Autodesk Fusion 360 part; units mm, degrees
(part 4 of 5)
sketch "Sketch2" plane through (0, 0, 0) normal (0, 0, 1) x (1, 0, 0) in component "spoilboard v12"
  arc A0 (1101.5761, 607.1637) -> (1101.5763, 647.1637) centre (1101.5762, 627.1637) ccw
  arc A1 (117.6237, 647.1637) -> (117.6239, 607.1637) centre (117.6238, 627.1637) ccw
  arc A2 (916.5761, 607.1637) -> (916.5763, 647.1637) centre (916.5762, 627.1637) ccw
  arc A3 (1036.0507, 647.1575) -> (1035.5361, 607.1642) centre (1036.0526, 627.1575) ccw
  line L0 (1016.0526, 627.1635) -> (1121.5762, 627.1635) construction
  line L1 (936.5762, 627.1635) -> (1016.0526, 627.1635) construction
  circle A4 centre (976.3144, 627.1635) radius 1.5875
  arc A5 (368.6639, 607.1642) -> (368.1493, 647.1575) centre (368.1474, 627.1575) ccw
  arc A6 (487.6237, 647.1637) -> (487.6239, 607.1637) centre (487.6238, 627.1637) ccw
  line L2 (97.6238, 627.1635) -> (388.1474, 627.1635) construction
  line L3 (467.6238, 627.1635) -> (936.5762, 627.1635) construction
  line L4 (388.1474, 627.1635) -> (467.6238, 627.1635) construction
  circle A7 centre (427.8856, 627.1635) radius 1.5875
  circle A8 centre (34.29, 1220) radius 17.145
  circle A9 centre (1184.91, 1220) radius 17.145
  circle A10 centre (897.255, 1220) radius 17.145
  circle A11 centre (609.6, 1220) radius 17.145
  line L5 (34.29, 1220) -> (626.745, 1220) construction
  line L6 (880.11, 1220) -> (1184.91, 1220) construction
  line L7 (626.745, 1220) -> (880.11, 1220) construction
  circle A12 centre (753.4275, 1220) radius 1.5875
  arc A13 (33.02, 1953.1525) -> (33.02, 1913.1525) centre (33.02, 1933.1525) ccw
  arc A14 (1186.18, 1913.1525) -> (1186.18, 1953.1525) centre (1186.18, 1933.1525) ccw
  arc A15 (461.4333, 1913.1525) -> (461.4333, 1953.1525) centre (461.4333, 1933.1525) ccw
  arc A16 (576.58, 1953.1525) -> (576.58, 1913.1525) centre (576.58, 1933.1525) ccw
  line L8 (33.02, 1933.1525) -> (481.4333, 1933.1525) construction
  line L9 (556.58, 1933.1525) -> (1186.18, 1933.1525) construction
  line L10 (481.4333, 1933.1525) -> (556.58, 1933.1525) construction
  circle A17 centre (519.0067, 1933.1525) radius 1.5875
  circle A18 centre (753.4275, 1220) radius 6
  circle A19 centre (976.3144, 627.1635) radius 6
  circle A20 centre (427.8856, 627.1635) radius 6
  circle A21 centre (519.0067, 1933.1525) radius 6
  arc A22 (117.6237, 1847.1637) -> (117.6239, 1807.1637) centre (117.6238, 1827.1637) ccw
  arc A23 (1101.5761, 1807.1637) -> (1101.5763, 1847.1637) centre (1101.5762, 1827.1637) ccw
  arc A24 (183.6639, 1807.1642) -> (183.1493, 1847.1575) centre (183.1474, 1827.1575) ccw
  arc A25 (302.6237, 1847.1637) -> (302.6239, 1807.1637) centre (302.6238, 1827.1637) ccw
  arc A26 (916.5761, 1807.1637) -> (916.5763, 1847.1637) centre (916.5762, 1827.1637) ccw
  arc A27 (1036.0507, 1847.1575) -> (1035.5361, 1807.1642) centre (1036.0526, 1827.1575) ccw
  line L11 (117.6238, 1827.1637) -> (203.1474, 1827.1637) construction
  line L12 (203.1474, 1827.1637) -> (282.6238, 1827.1637) construction
  line L13 (282.6238, 1827.1637) -> (936.5762, 1827.1637) construction
  line L14 (1016.0526, 1827.1637) -> (1101.5762, 1827.1637) construction
  line L15 (936.5762, 1827.1637) -> (1016.0526, 1827.1637) construction
  circle A28 centre (242.8856, 1827.1637) radius 1.5875
  circle A29 centre (976.3144, 1827.1637) radius 1.5875
  circle A30 centre (242.8856, 1827.1637) radius 6
  circle A31 centre (976.3144, 1827.1637) radius 6
  arc A32 (33.02, 933.1525) -> (33.02, 893.1525) centre (33.02, 913.1525) ccw
  arc A33 (1186.18, 893.1525) -> (1186.18, 933.1525) centre (1186.18, 913.1525) ccw
  arc A34 (99.06, 893.1525) -> (99.06, 933.1525) centre (99.06, 913.1525) ccw
  arc A35 (214.2067, 933.1525) -> (214.2067, 893.1525) centre (214.2067, 913.1525) ccw
  arc A36 (1004.9933, 893.1525) -> (1004.9933, 933.1525) centre (1004.9933, 913.1525) ccw
  arc A37 (1120.14, 933.1525) -> (1120.14, 893.1525) centre (1120.14, 913.1525) ccw
  line L16 (33.02, 913.1525) -> (119.06, 913.1525) construction
  line L17 (119.06, 913.1525) -> (194.2067, 913.1525) construction
  line L18 (194.2067, 913.1525) -> (1024.9933, 913.1525) construction
  line L19 (1100.14, 913.1525) -> (1186.18, 913.1525) construction
  line L20 (1024.9933, 913.1525) -> (1100.14, 913.1525) construction
  circle A38 centre (156.6333, 913.1525) radius 1.5875
  circle A39 centre (156.6333, 913.1525) radius 6
  circle A40 centre (1062.5667, 913.1525) radius 1.5875
  circle A41 centre (1062.5667, 913.1525) radius 6
  line L21 (1191.9077, 14.92) -> (1177.9123, 14.92)
  arc A42 (1191.9077, 14.92) -> (1191.9077, 25.08) centre (1191.9077, 20) ccw
  line L22 (1177.9123, 25.08) -> (1191.9077, 25.08)
  arc A43 (1177.9123, 25.08) -> (1177.9123, 14.92) centre (1177.9123, 20) ccw
  line L23 (1191.9077, 2414.92) -> (1177.9123, 2414.92)
  arc A44 (1191.9077, 2414.92) -> (1191.9077, 2425.08) centre (1191.9077, 2420) ccw
  line L24 (1177.9123, 2425.08) -> (1191.9077, 2425.08)
  arc A45 (1177.9123, 2425.08) -> (1177.9123, 2414.92) centre (1177.9123, 2420) ccw
  line L25 (1177.9123, 2420) -> (1191.9077, 2420) construction
  line L26 (1177.9123, 20) -> (1191.9077, 20) construction
  line L27 (1184.91, 20) -> (1184.91, 2420) construction
  arc A46 (1101.5761, 207.1637) -> (1101.5763, 247.1637) centre (1101.5762, 227.1637) ccw
  line L28 (1101.5762, 227.1637) -> (1300, 227.1637) construction
  circle A47 centre (1184.91, 227.1637) radius 1.5875
  circle A48 centre (1184.91, 227.1637) radius 6
  dimension "d143" = 3.175
  dimension "d144" = 3.175
  dimension "d145" = 3.175
  dimension "d146" = 3.175
  dimension "d148" = 12
  dimension "d149" = 12
  dimension "d150" = 12
  dimension "d151" = 12
  dimension "d157" = 3.175
  dimension "d158" = 3.175
  dimension "d159" = 12
  dimension "d160" = 12
  dimension "d161" = 3.175
  dimension "d162" = 12
  dimension "d163" = 3.175
  dimension "d164" = 12
  dimension "d165" = 3.175
  dimension "d166" = 12
  constraint horizontal L2
  constraint midpoint L0.end A0
  constraint midpoint L2.start A1
  constraint coincident A2 L1.start
  constraint coincident A3 L0.start
  constraint midpoint L1 A4.centre
  constraint coincident A5 L2.end
  constraint coincident A6 L3.start
  constraint midpoint L4 A7.centre
  constraint coincident A8.centre L5.start
  constraint coincident A9.centre L6.end
  constraint coincident A11 L5.end
  constraint coincident A10 L6.start
  constraint midpoint L7 A12.centre
  constraint coincident A13.centre L8.start
  constraint coincident A14.centre L9.end
  constraint coincident A15 L8.end
  constraint coincident A16 L9.start
  constraint midpoint L10 A17.centre
  constraint concentric A12 A18
  constraint concentric A4 A19
  constraint concentric A7 A20
  constraint concentric A17 A21
  constraint coincident A22.centre L11.start
  constraint coincident A23.centre L14.end
  constraint coincident A24 L11.end
  constraint coincident A25 L12.end
  constraint coincident A26 L13.end
  constraint coincident A27 L14.start
  constraint midpoint L12 A28.centre
  constraint midpoint L15 A29.centre
  constraint concentric A28 A30
  constraint concentric A29 A31
  constraint coincident A32.centre L16.start
  constraint coincident A33.centre L19.end
  constraint coincident A34 L16.end
  constraint coincident A35 L17.end
  constraint coincident A36 L18.end
  constraint coincident A37 L19.start
  constraint midpoint L17 A38.centre
  constraint concentric A38 A39
  constraint midpoint L20 A40.centre
  constraint concentric A40 A41
  constraint coincident A45.centre L25.start
  constraint coincident A44.centre L25.end
  constraint coincident A43.centre L26.start
  constraint coincident A42.centre L26.end
  constraint midpoint L26 L27.start
  constraint midpoint L25 L27.end
  constraint coincident A46.centre L28.start
  constraint horizontal L28
  constraint coincident L28 A47.centre
  constraint coincident L27 A47.centre
  constraint concentric A47 A48
  measures "d143" diameter of A4
  measures "d144" diameter of A7
  measures "d145" diameter of A12
  measures "d146" diameter of A17
  measures "d148" diameter of A18
  measures "d149" diameter of A19
  measures "d150" diameter of A20
  measures "d151" diameter of A21
  measures "d157" diameter of A28
  measures "d158" diameter of A29
  measures "d159" diameter of A30
  measures "d160" diameter of A31
  measures "d161" diameter of A38
  measures "d162" diameter of A39
  measures "d163" diameter of A40
  measures "d164" diameter of A41
  measures "d165" diameter of A47
  measures "d166" diameter of A48
extrude "Extrude8" [suppressed] in component "SpoilBoard"
extrude "Extrude9" [suppressed] in component "SpoilBoard"
sketch "Sketch3" plane through (0, 0, 19.05) normal (0, 0, 1) x (-1, 0, 0) in component "spoilboard v12"
  circle A0 centre (-753.4275, -1220) radius 6
  circle A1 centre (-427.8856, -627.1635) radius 6
  circle A2 centre (-976.3144, -627.1635) radius 6
  circle A3 centre (-165.1, -965.2) radius 9.525
  circle A4 centre (-165.1, -1765.3) radius 9.525
  circle A5 centre (-165.1, -165.1) radius 9.525
  circle A6 centre (-165.1, -2286) radius 9.525
  circle A7 centre (-257.175, -22.225) radius 3.175
  circle A8 centre (-1019.175, -22.225) radius 3.175
  line L0 (-666.0507, -2247.1575) -> (-731.5763, -2247.1637)
  arc A9 (-731.5761, -2207.1637) -> (-731.5763, -2247.1637) centre (-731.5762, -2227.1637) ccw
  line L1 (-731.5761, -2207.1637) -> (-665.5361, -2207.1642)
  arc A10 (-666.0507, -2247.1575) -> (-665.5361, -2207.1642) centre (-666.0526, -2227.1575) ccw
  line L2 (-1036.0507, -1847.1575) -> (-1101.5763, -1847.1637)
  arc A11 (-1101.5761, -1807.1637) -> (-1101.5763, -1847.1637) centre (-1101.5762, -1827.1637) ccw
  line L3 (-1101.5761, -1807.1637) -> (-1035.5361, -1807.1642)
  arc A12 (-1036.0507, -1847.1575) -> (-1035.5361, -1807.1642) centre (-1036.0526, -1827.1575) ccw
  line L4 (-368.6639, -1807.1642) -> (-302.6239, -1807.1637)
  arc A13 (-302.6237, -1847.1637) -> (-302.6239, -1807.1637) centre (-302.6238, -1827.1637) ccw
  line L5 (-302.6237, -1847.1637) -> (-368.1493, -1847.1575)
  arc A14 (-368.6639, -1807.1642) -> (-368.1493, -1847.1575) centre (-368.1474, -1827.1575) ccw
  line L6 (-666.0507, -1447.1575) -> (-731.5763, -1447.1637)
  arc A15 (-731.5761, -1407.1637) -> (-731.5763, -1447.1637) centre (-731.5762, -1427.1637) ccw
  line L7 (-731.5761, -1407.1637) -> (-665.5361, -1407.1642)
  arc A16 (-666.0507, -1447.1575) -> (-665.5361, -1407.1642) centre (-666.0526, -1427.1575) ccw
  line L8 (-1101.5761, -207.1637) -> (-1035.5361, -207.1642)
  arc A17 (-1036.0507, -247.1575) -> (-1035.5361, -207.1642) centre (-1036.0526, -227.1575) ccw
  line L9 (-1036.0507, -247.1575) -> (-1101.5763, -247.1637)
  arc A18 (-1101.5761, -207.1637) -> (-1101.5763, -247.1637) centre (-1101.5762, -227.1637) ccw
  line L10 (-368.6639, -207.1642) -> (-302.6239, -207.1637)
  arc A19 (-302.6237, -247.1637) -> (-302.6239, -207.1637) centre (-302.6238, -227.1637) ccw
  line L11 (-302.6237, -247.1637) -> (-368.1493, -247.1575)
  arc A20 (-368.6639, -207.1642) -> (-368.1493, -247.1575) centre (-368.1474, -227.1575) ccw
  line L12 (-553.6639, -607.1642) -> (-487.6239, -607.1637)
  arc A21 (-487.6237, -647.1637) -> (-487.6239, -607.1637) centre (-487.6238, -627.1637) ccw
  line L13 (-487.6237, -647.1637) -> (-553.1493, -647.1575)
  arc A22 (-553.6639, -607.1642) -> (-553.1493, -647.1575) centre (-553.1474, -627.1575) ccw
  line L14 (-1036.0507, -1047.1575) -> (-1101.5763, -1047.1637)
  arc A23 (-1101.5761, -1007.1637) -> (-1101.5763, -1047.1637) centre (-1101.5762, -1027.1637) ccw
  line L15 (-1101.5761, -1007.1637) -> (-1035.5361, -1007.1642)
  arc A24 (-1036.0507, -1047.1575) -> (-1035.5361, -1007.1642) centre (-1036.0526, -1027.1575) ccw
  line L16 (-368.6639, -1007.1642) -> (-302.6239, -1007.1637)
  arc A25 (-302.6237, -1047.1637) -> (-302.6239, -1007.1637) centre (-302.6238, -1027.1637) ccw
  line L17 (-302.6237, -1047.1637) -> (-368.1493, -1047.1575)
  arc A26 (-368.6639, -1007.1642) -> (-368.1493, -1047.1575) centre (-368.1474, -1027.1575) ccw
  line L18 (-99.06, -2093.1525) -> (-33.02, -2093.1525)
  arc A27 (-33.02, -2133.1525) -> (-33.02, -2093.1525) centre (-33.02, -2113.1525) ccw
  line L19 (-33.02, -2133.1525) -> (-99.06, -2133.1525)
  arc A28 (-99.06, -2093.1525) -> (-99.06, -2133.1525) centre (-99.06, -2113.1525) ccw
  arc A29 (-461.4333, -1693.1525) -> (-461.4333, -1733.1525) centre (-461.4333, -1713.1525) ccw
  line L20 (-461.4333, -1693.1525) -> (-395.3933, -1693.1525)
  arc A30 (-395.3933, -1733.1525) -> (-395.3933, -1693.1525) centre (-395.3933, -1713.1525) ccw
  line L21 (-395.3933, -1733.1525) -> (-461.4333, -1733.1525)
  line L22 (-99.06, -1913.1525) -> (-33.02, -1913.1525)
  arc A31 (-33.02, -1953.1525) -> (-33.02, -1913.1525) centre (-33.02, -1933.1525) ccw
  line L23 (-33.02, -1953.1525) -> (-99.06, -1953.1525)
  arc A32 (-99.06, -1913.1525) -> (-99.06, -1953.1525) centre (-99.06, -1933.1525) ccw
  line L24 (-99.06, -1293.1525) -> (-33.02, -1293.1525)
  arc A33 (-33.02, -1333.1525) -> (-33.02, -1293.1525) centre (-33.02, -1313.1525) ccw
  line L25 (-33.02, -1333.1525) -> (-99.06, -1333.1525)
  arc A34 (-99.06, -1293.1525) -> (-99.06, -1333.1525) centre (-99.06, -1313.1525) ccw
  arc A35 (-642.62, -2093.1525) -> (-642.62, -2133.1525) centre (-642.62, -2113.1525) ccw
  line L26 (-642.62, -2093.1525) -> (-576.58, -2093.1525)
  arc A36 (-576.58, -2133.1525) -> (-576.58, -2093.1525) centre (-576.58, -2113.1525) ccw
  line L27 (-576.58, -2133.1525) -> (-642.62, -2133.1525)
  arc A37 (-642.62, -2313.1525) -> (-642.62, -2353.1525) centre (-642.62, -2333.1525) ccw
  line L28 (-642.62, -2313.1525) -> (-576.58, -2313.1525)
  arc A38 (-576.58, -2353.1525) -> (-576.58, -2313.1525) centre (-576.58, -2333.1525) ccw
  line L29 (-576.58, -2353.1525) -> (-642.62, -2353.1525)
  arc A39 (-642.62, -1693.1525) -> (-642.62, -1733.1525) centre (-642.62, -1713.1525) ccw
  line L30 (-642.62, -1693.1525) -> (-576.58, -1693.1525)
  arc A40 (-576.58, -1733.1525) -> (-576.58, -1693.1525) centre (-576.58, -1713.1525) ccw
  line L31 (-576.58, -1733.1525) -> (-642.62, -1733.1525)
  arc A41 (-642.62, -1913.1525) -> (-642.62, -1953.1525) centre (-642.62, -1933.1525) ccw
  line L32 (-642.62, -1913.1525) -> (-576.58, -1913.1525)
  arc A42 (-576.58, -1953.1525) -> (-576.58, -1913.1525) centre (-576.58, -1933.1525) ccw
  line L33 (-576.58, -1953.1525) -> (-642.62, -1953.1525)
  arc A43 (-642.62, -1293.1525) -> (-642.62, -1333.1525) centre (-642.62, -1313.1525) ccw
  line L34 (-642.62, -1293.1525) -> (-576.58, -1293.1525)
  arc A44 (-576.58, -1333.1525) -> (-576.58, -1293.1525) centre (-576.58, -1313.1525) ccw
  line L35 (-576.58, -1333.1525) -> (-642.62, -1333.1525)
  arc A45 (-642.62, -1513.1525) -> (-642.62, -1553.1525) centre (-642.62, -1533.1525) ccw
  line L36 (-642.62, -1513.1525) -> (-576.58, -1513.1525)
  arc A46 (-576.58, -1553.1525) -> (-576.58, -1513.1525) centre (-576.58, -1533.1525) ccw
  line L37 (-576.58, -1553.1525) -> (-642.62, -1553.1525)
  line L38 (-33.02, -133.1525) -> (-99.06, -133.1525)
  arc A47 (-99.06, -93.1525) -> (-99.06, -133.1525) centre (-99.06, -113.1525) ccw
  line L39 (-99.06, -93.1525) -> (-33.02, -93.1525)
  arc A48 (-33.02, -133.1525) -> (-33.02, -93.1525) centre (-33.02, -113.1525) ccw
  line L40 (-214.2067, -353.1525) -> (-280.2467, -353.1525)
  arc A49 (-280.2467, -313.1525) -> (-280.2467, -353.1525) centre (-280.2467, -333.1525) ccw
  line L41 (-280.2467, -313.1525) -> (-214.2067, -313.1525)
  arc A50 (-214.2067, -353.1525) -> (-214.2067, -313.1525) centre (-214.2067, -333.1525) ccw
  arc A51 (-461.4333, -713.1525) -> (-461.4333, -753.1525) centre (-461.4333, -733.1525) ccw
  line L42 (-461.4333, -713.1525) -> (-395.3933, -713.1525)
  arc A52 (-395.3933, -753.1525) -> (-395.3933, -713.1525) centre (-395.3933, -733.1525) ccw
  line L43 (-395.3933, -753.1525) -> (-461.4333, -753.1525)
  arc A53 (-280.2467, -1113.1525) -> (-280.2467, -1153.1525) centre (-280.2467, -1133.1525) ccw
  line L44 (-280.2467, -1113.1525) -> (-214.2067, -1113.1525)
  arc A54 (-214.2067, -1153.1525) -> (-214.2067, -1113.1525) centre (-214.2067, -1133.1525) ccw
  line L45 (-214.2067, -1153.1525) -> (-280.2467, -1153.1525)
  line L46 (-280.2467, -893.1525) -> (-214.2067, -893.1525)
  arc A55 (-214.2067, -933.1525) -> (-214.2067, -893.1525) centre (-214.2067, -913.1525) ccw
  line L47 (-214.2067, -933.1525) -> (-280.2467, -933.1525)
  arc A56 (-280.2467, -893.1525) -> (-280.2467, -933.1525) centre (-280.2467, -913.1525) ccw
  line L48 (-1120.14, -133.1525) -> (-1186.18, -133.1525)
  arc A57 (-1186.18, -93.1525) -> (-1186.18, -133.1525) centre (-1186.18, -113.1525) ccw
  line L49 (-1186.18, -93.1525) -> (-1120.14, -93.1525)
  arc A58 (-1120.14, -133.1525) -> (-1120.14, -93.1525) centre (-1120.14, -113.1525) ccw
  line L50 (-1120.14, -353.1525) -> (-1186.18, -353.1525)
  arc A59 (-1186.18, -313.1525) -> (-1186.18, -353.1525) centre (-1186.18, -333.1525) ccw
  line L51 (-1186.18, -313.1525) -> (-1120.14, -313.1525)
  arc A60 (-1120.14, -353.1525) -> (-1120.14, -313.1525) centre (-1120.14, -333.1525) ccw
  arc A61 (-642.62, -713.1525) -> (-642.62, -753.1525) centre (-642.62, -733.1525) ccw
  line L52 (-642.62, -713.1525) -> (-576.58, -713.1525)
  arc A62 (-576.58, -753.1525) -> (-576.58, -713.1525) centre (-576.58, -733.1525) ccw
  line L53 (-576.58, -753.1525) -> (-642.62, -753.1525)
  arc A63 (-642.62, -493.1525) -> (-642.62, -533.1525) centre (-642.62, -513.1525) ccw
  line L54 (-642.62, -493.1525) -> (-576.58, -493.1525)
  arc A64 (-576.58, -533.1525) -> (-576.58, -493.1525) centre (-576.58, -513.1525) ccw
  line L55 (-576.58, -533.1525) -> (-642.62, -533.1525)
  arc A65 (-642.62, -1113.1525) -> (-642.62, -1153.1525) centre (-642.62, -1133.1525) ccw
  line L56 (-642.62, -1113.1525) -> (-576.58, -1113.1525)
  arc A66 (-576.58, -1153.1525) -> (-576.58, -1113.1525) centre (-576.58, -1133.1525) ccw
  line L57 (-576.58, -1153.1525) -> (-642.62, -1153.1525)
  arc A67 (-642.62, -893.1525) -> (-642.62, -933.1525) centre (-642.62, -913.1525) ccw
  line L58 (-642.62, -893.1525) -> (-576.58, -893.1525)
  arc A68 (-576.58, -933.1525) -> (-576.58, -893.1525) centre (-576.58, -913.1525) ccw
  line L59 (-576.58, -933.1525) -> (-642.62, -933.1525)
  line L60 (-757.7667, -933.1525) -> (-823.8067, -933.1525)
  arc A69 (-823.8067, -893.1525) -> (-823.8067, -933.1525) centre (-823.8067, -913.1525) ccw
  line L61 (-823.8067, -893.1525) -> (-757.7667, -893.1525)
  arc A70 (-757.7667, -933.1525) -> (-757.7667, -893.1525) centre (-757.7667, -913.1525) ccw
  line L62 (-757.7667, -1153.1525) -> (-823.8067, -1153.1525)
  arc A71 (-823.8067, -1113.1525) -> (-823.8067, -1153.1525) centre (-823.8067, -1133.1525) ccw
  line L63 (-823.8067, -1113.1525) -> (-757.7667, -1113.1525)
  arc A72 (-757.7667, -1153.1525) -> (-757.7667, -1113.1525) centre (-757.7667, -1133.1525) ccw
  line L64 (-757.7667, -533.1525) -> (-823.8067, -533.1525)
  arc A73 (-823.8067, -493.1525) -> (-823.8067, -533.1525) centre (-823.8067, -513.1525) ccw
  line L65 (-823.8067, -493.1525) -> (-757.7667, -493.1525)
  arc A74 (-757.7667, -533.1525) -> (-757.7667, -493.1525) centre (-757.7667, -513.1525) ccw
  line L66 (-757.7667, -753.1525) -> (-823.8067, -753.1525)
  arc A75 (-823.8067, -713.1525) -> (-823.8067, -753.1525) centre (-823.8067, -733.1525) ccw
  line L67 (-823.8067, -713.1525) -> (-757.7667, -713.1525)
  arc A76 (-757.7667, -753.1525) -> (-757.7667, -713.1525) centre (-757.7667, -733.1525) ccw
  line L68 (-938.9533, -353.1525) -> (-1004.9933, -353.1525)
  arc A77 (-1004.9933, -313.1525) -> (-1004.9933, -353.1525) centre (-1004.9933, -333.1525) ccw
  line L69 (-1004.9933, -313.1525) -> (-938.9533, -313.1525)
  arc A78 (-938.9533, -353.1525) -> (-938.9533, -313.1525) centre (-938.9533, -333.1525) ccw
  line L70 (-938.9533, -133.1525) -> (-1004.9933, -133.1525)
  arc A79 (-1004.9933, -93.1525) -> (-1004.9933, -133.1525) centre (-1004.9933, -113.1525) ccw
  line L71 (-1004.9933, -93.1525) -> (-938.9533, -93.1525)
  arc A80 (-938.9533, -133.1525) -> (-938.9533, -93.1525) centre (-938.9533, -113.1525) ccw
  line L72 (-99.06, -893.1525) -> (-33.02, -893.1525)
  arc A81 (-33.02, -933.1525) -> (-33.02, -893.1525) centre (-33.02, -913.1525) ccw
  line L73 (-33.02, -933.1525) -> (-99.06, -933.1525)
  arc A82 (-99.06, -893.1525) -> (-99.06, -933.1525) centre (-99.06, -913.1525) ccw
  arc A83 (-461.4333, -493.1525) -> (-461.4333, -533.1525) centre (-461.4333, -513.1525) ccw
  line L74 (-461.4333, -493.1525) -> (-395.3933, -493.1525)
  arc A84 (-395.3933, -533.1525) -> (-395.3933, -493.1525) centre (-395.3933, -513.1525) ccw
  line L75 (-395.3933, -533.1525) -> (-461.4333, -533.1525)
  line L76 (-99.06, -713.1525) -> (-33.02, -713.1525)
  arc A85 (-33.02, -753.1525) -> (-33.02, -713.1525) centre (-33.02, -733.1525) ccw
  line L77 (-33.02, -753.1525) -> (-99.06, -753.1525)
  arc A86 (-99.06, -713.1525) -> (-99.06, -753.1525) centre (-99.06, -733.1525) ccw
  line L78 (-33.02, -353.1525) -> (-99.06, -353.1525)
  arc A87 (-99.06, -313.1525) -> (-99.06, -353.1525) centre (-99.06, -333.1525) ccw
  line L79 (-99.06, -313.1525) -> (-33.02, -313.1525)
  arc A88 (-33.02, -353.1525) -> (-33.02, -313.1525) centre (-33.02, -333.1525) ccw
  line L80 (-1186.18, -1513.1525) -> (-1120.14, -1513.1525)
  arc A89 (-1120.14, -1553.1525) -> (-1120.14, -1513.1525) centre (-1120.14, -1533.1525) ccw
  line L81 (-1120.14, -1553.1525) -> (-1186.18, -1553.1525)
  arc A90 (-1186.18, -1513.1525) -> (-1186.18, -1553.1525) centre (-1186.18, -1533.1525) ccw
  line L82 (-1120.14, -1333.1525) -> (-1186.18, -1333.1525)
  arc A91 (-1186.18, -1293.1525) -> (-1186.18, -1333.1525) centre (-1186.18, -1313.1525) ccw
  line L83 (-1186.18, -1293.1525) -> (-1120.14, -1293.1525)
  arc A92 (-1120.14, -1333.1525) -> (-1120.14, -1293.1525) centre (-1120.14, -1313.1525) ccw
  line L84 (-1186.18, -1913.1525) -> (-1120.14, -1913.1525)
  arc A93 (-1120.14, -1953.1525) -> (-1120.14, -1913.1525) centre (-1120.14, -1933.1525) ccw
  line L85 (-1120.14, -1953.1525) -> (-1186.18, -1953.1525)
  arc A94 (-1186.18, -1913.1525) -> (-1186.18, -1953.1525) centre (-1186.18, -1933.1525) ccw
  line L86 (-1120.14, -1733.1525) -> (-1186.18, -1733.1525)
  arc A95 (-1186.18, -1693.1525) -> (-1186.18, -1733.1525) centre (-1186.18, -1713.1525) ccw
  line L87 (-1186.18, -1693.1525) -> (-1120.14, -1693.1525)
  arc A96 (-1120.14, -1733.1525) -> (-1120.14, -1693.1525) centre (-1120.14, -1713.1525) ccw
  line L88 (-1186.18, -2313.1525) -> (-1120.14, -2313.1525)
  arc A97 (-1120.14, -2353.1525) -> (-1120.14, -2313.1525) centre (-1120.14, -2333.1525) ccw
  line L89 (-1120.14, -2353.1525) -> (-1186.18, -2353.1525)
  arc A98 (-1186.18, -2313.1525) -> (-1186.18, -2353.1525) centre (-1186.18, -2333.1525) ccw
  line L90 (-1120.14, -2133.1525) -> (-1186.18, -2133.1525)
  arc A99 (-1186.18, -2093.1525) -> (-1186.18, -2133.1525) centre (-1186.18, -2113.1525) ccw
  line L91 (-1186.18, -2093.1525) -> (-1120.14, -2093.1525)
  arc A100 (-1120.14, -2133.1525) -> (-1120.14, -2093.1525) centre (-1120.14, -2113.1525) ccw
  arc A101 (-280.2467, -1513.1525) -> (-280.2467, -1553.1525) centre (-280.2467, -1533.1525) ccw
  line L92 (-280.2467, -1513.1525) -> (-214.2067, -1513.1525)
  arc A102 (-214.2067, -1553.1525) -> (-214.2067, -1513.1525) centre (-214.2067, -1533.1525) ccw
  line L93 (-214.2067, -1553.1525) -> (-280.2467, -1553.1525)
  line L94 (-280.2467, -1293.1525) -> (-214.2067, -1293.1525)
  arc A103 (-214.2067, -1333.1525) -> (-214.2067, -1293.1525) centre (-214.2067, -1313.1525) ccw
  line L95 (-214.2067, -1333.1525) -> (-280.2467, -1333.1525)
  arc A104 (-280.2467, -1293.1525) -> (-280.2467, -1333.1525) centre (-280.2467, -1313.1525) ccw
  arc A105 (-461.4333, -1913.1525) -> (-461.4333, -1953.1525) centre (-461.4333, -1933.1525) ccw
  line L96 (-461.4333, -1913.1525) -> (-395.3933, -1913.1525)
  arc A106 (-395.3933, -1953.1525) -> (-395.3933, -1913.1525) centre (-395.3933, -1933.1525) ccw
  line L97 (-395.3933, -1953.1525) -> (-461.4333, -1953.1525)
  arc A107 (-280.2467, -2313.1525) -> (-280.2467, -2353.1525) centre (-280.2467, -2333.1525) ccw
  line L98 (-280.2467, -2313.1525) -> (-214.2067, -2313.1525)
  arc A108 (-214.2067, -2353.1525) -> (-214.2067, -2313.1525) centre (-214.2067, -2333.1525) ccw
  line L99 (-214.2067, -2353.1525) -> (-280.2467, -2353.1525)
  line L100 (-280.2467, -2093.1525) -> (-214.2067, -2093.1525)
  arc A109 (-214.2067, -2133.1525) -> (-214.2067, -2093.1525) centre (-214.2067, -2113.1525) ccw
  line L101 (-214.2067, -2133.1525) -> (-280.2467, -2133.1525)
  arc A110 (-280.2467, -2093.1525) -> (-280.2467, -2133.1525) centre (-280.2467, -2113.1525) ccw
  line L102 (-553.6639, -1007.1642) -> (-487.6239, -1007.1637)
  arc A111 (-487.6237, -1047.1637) -> (-487.6239, -1007.1637) centre (-487.6238, -1027.1637) ccw
  line L103 (-487.6237, -1047.1637) -> (-553.1493, -1047.1575)
  arc A112 (-553.6639, -1007.1642) -> (-553.1493, -1047.1575) centre (-553.1474, -1027.1575) ccw
  line L104 (-1036.0507, -647.1575) -> (-1101.5763, -647.1637)
  arc A113 (-1101.5761, -607.1637) -> (-1101.5763, -647.1637) centre (-1101.5762, -627.1637) ccw
  line L105 (-1101.5761, -607.1637) -> (-1035.5361, -607.1642)
  arc A114 (-1036.0507, -647.1575) -> (-1035.5361, -607.1642) centre (-1036.0526, -627.1575) ccw
  line L106 (-368.6639, -607.1642) -> (-302.6239, -607.1637)
  arc A115 (-302.6237, -647.1637) -> (-302.6239, -607.1637) centre (-302.6238, -627.1637) ccw
  line L107 (-302.6237, -647.1637) -> (-368.1493, -647.1575)
  arc A116 (-368.6639, -607.1642) -> (-368.1493, -647.1575) centre (-368.1474, -627.1575) ccw
  line L108 (-553.6639, -207.1642) -> (-487.6239, -207.1637)
  arc A117 (-487.6237, -247.1637) -> (-487.6239, -207.1637) centre (-487.6238, -227.1637) ccw
  line L109 (-487.6237, -247.1637) -> (-553.1493, -247.1575)
  arc A118 (-553.6639, -207.1642) -> (-553.1493, -247.1575) centre (-553.1474, -227.1575) ccw
  line L110 (-183.6639, -1407.1642) -> (-117.6239, -1407.1637)
  arc A119 (-117.6237, -1447.1637) -> (-117.6239, -1407.1637) centre (-117.6238, -1427.1637) ccw
  line L111 (-117.6237, -1447.1637) -> (-183.1493, -1447.1575)
  arc A120 (-183.6639, -1407.1642) -> (-183.1493, -1447.1575) centre (-183.1474, -1427.1575) ccw
  arc A121 (-916.5761, -1407.1637) -> (-916.5763, -1447.1637) centre (-916.5762, -1427.1637) ccw
  line L112 (-916.5761, -1407.1637) -> (-850.5361, -1407.1642)
  arc A122 (-851.0507, -1447.1575) -> (-850.5361, -1407.1642) centre (-851.0526, -1427.1575) ccw
  line L113 (-851.0507, -1447.1575) -> (-916.5763, -1447.1637)
  line L114 (-553.6639, -1807.1642) -> (-487.6239, -1807.1637)
  arc A123 (-487.6237, -1847.1637) -> (-487.6239, -1807.1637) centre (-487.6238, -1827.1637) ccw
  line L115 (-487.6237, -1847.1637) -> (-553.1493, -1847.1575)
  arc A124 (-553.6639, -1807.1642) -> (-553.1493, -1847.1575) centre (-553.1474, -1827.1575) ccw
  line L116 (-183.6639, -2207.1642) -> (-117.6239, -2207.1637)
  arc A125 (-117.6237, -2247.1637) -> (-117.6239, -2207.1637) centre (-117.6238, -2227.1637) ccw
  line L117 (-117.6237, -2247.1637) -> (-183.1493, -2247.1575)
  arc A126 (-183.6639, -2207.1642) -> (-183.1493, -2247.1575) centre (-183.1474, -2227.1575) ccw
  arc A127 (-916.5761, -2207.1637) -> (-916.5763, -2247.1637) centre (-916.5762, -2227.1637) ccw
  line L118 (-916.5761, -2207.1637) -> (-850.5361, -2207.1642)
  arc A128 (-851.0507, -2247.1575) -> (-850.5361, -2207.1642) centre (-851.0526, -2227.1575) ccw
  line L119 (-851.0507, -2247.1575) -> (-916.5763, -2247.1637)
  line L120 (-553.6639, -2207.1642) -> (-487.6239, -2207.1637)
  arc A129 (-487.6237, -2247.1637) -> (-487.6239, -2207.1637) centre (-487.6238, -2227.1637) ccw
  line L121 (-487.6237, -2247.1637) -> (-553.1493, -2247.1575)
  arc A130 (-553.6639, -2207.1642) -> (-553.1493, -2247.1575) centre (-553.1474, -2227.1575) ccw
  arc A131 (-916.5761, -1807.1637) -> (-916.5763, -1847.1637) centre (-916.5762, -1827.1637) ccw
  line L122 (-916.5761, -1807.1637) -> (-850.5361, -1807.1642)
  arc A132 (-851.0507, -1847.1575) -> (-850.5361, -1807.1642) centre (-851.0526, -1827.1575) ccw
  line L123 (-851.0507, -1847.1575) -> (-916.5763, -1847.1637)
  line L124 (-183.6639, -1807.1642) -> (-117.6239, -1807.1637)
  arc A133 (-117.6237, -1847.1637) -> (-117.6239, -1807.1637) centre (-117.6238, -1827.1637) ccw
  line L125 (-117.6237, -1847.1637) -> (-183.1493, -1847.1575)
  arc A134 (-183.6639, -1807.1642) -> (-183.1493, -1847.1575) centre (-183.1474, -1827.1575) ccw
  line L126 (-553.6639, -1407.1642) -> (-487.6239, -1407.1637)
  arc A135 (-487.6237, -1447.1637) -> (-487.6239, -1407.1637) centre (-487.6238, -1427.1637) ccw
  line L127 (-487.6237, -1447.1637) -> (-553.1493, -1447.1575)
  arc A136 (-553.6639, -1407.1642) -> (-553.1493, -1447.1575) centre (-553.1474, -1427.1575) ccw
  line L128 (-916.5761, -207.1637) -> (-850.5361, -207.1642)
  arc A137 (-851.0507, -247.1575) -> (-850.5361, -207.1642) centre (-851.0526, -227.1575) ccw
  line L129 (-851.0507, -247.1575) -> (-916.5763, -247.1637)
  arc A138 (-916.5761, -207.1637) -> (-916.5763, -247.1637) centre (-916.5762, -227.1637) ccw
  line L130 (-183.6639, -207.1642) -> (-117.6239, -207.1637)
  arc A139 (-117.6237, -247.1637) -> (-117.6239, -207.1637) centre (-117.6238, -227.1637) ccw
  line L131 (-117.6237, -247.1637) -> (-183.1493, -247.1575)
  arc A140 (-183.6639, -207.1642) -> (-183.1493, -247.1575) centre (-183.1474, -227.1575) ccw
  line L132 (-666.0507, -647.1575) -> (-731.5763, -647.1637)
  arc A141 (-731.5761, -607.1637) -> (-731.5763, -647.1637) centre (-731.5762, -627.1637) ccw
  line L133 (-731.5761, -607.1637) -> (-665.5361, -607.1642)
  arc A142 (-666.0507, -647.1575) -> (-665.5361, -607.1642) centre (-666.0526, -627.1575) ccw
  arc A143 (-916.5761, -1007.1637) -> (-916.5763, -1047.1637) centre (-916.5762, -1027.1637) ccw
  line L134 (-916.5761, -1007.1637) -> (-850.5361, -1007.1642)
  arc A144 (-851.0507, -1047.1575) -> (-850.5361, -1007.1642) centre (-851.0526, -1027.1575) ccw
  line L135 (-851.0507, -1047.1575) -> (-916.5763, -1047.1637)
  line L136 (-183.6639, -1007.1642) -> (-117.6239, -1007.1637)
  arc A145 (-117.6237, -1047.1637) -> (-117.6239, -1007.1637) centre (-117.6238, -1027.1637) ccw
  line L137 (-117.6237, -1047.1637) -> (-183.1493, -1047.1575)
  arc A146 (-183.6639, -1007.1642) -> (-183.1493, -1047.1575) centre (-183.1474, -1027.1575) ccw
  arc A147 (-461.4333, -2313.1525) -> (-461.4333, -2353.1525) centre (-461.4333, -2333.1525) ccw
  line L138 (-461.4333, -2313.1525) -> (-395.3933, -2313.1525)
  arc A148 (-395.3933, -2353.1525) -> (-395.3933, -2313.1525) centre (-395.3933, -2333.1525) ccw
  line L139 (-395.3933, -2353.1525) -> (-461.4333, -2353.1525)
  line L140 (-280.2467, -1693.1525) -> (-214.2067, -1693.1525)
  arc A149 (-214.2067, -1733.1525) -> (-214.2067, -1693.1525) centre (-214.2067, -1713.1525) ccw
  line L141 (-214.2067, -1733.1525) -> (-280.2467, -1733.1525)
  arc A150 (-280.2467, -1693.1525) -> (-280.2467, -1733.1525) centre (-280.2467, -1713.1525) ccw
  arc A151 (-280.2467, -1913.1525) -> (-280.2467, -1953.1525) centre (-280.2467, -1933.1525) ccw
  line L142 (-280.2467, -1913.1525) -> (-214.2067, -1913.1525)
  arc A152 (-214.2067, -1953.1525) -> (-214.2067, -1913.1525) centre (-214.2067, -1933.1525) ccw
  line L143 (-214.2067, -1953.1525) -> (-280.2467, -1953.1525)
  arc A153 (-461.4333, -1513.1525) -> (-461.4333, -1553.1525) centre (-461.4333, -1533.1525) ccw
  line L144 (-461.4333, -1513.1525) -> (-395.3933, -1513.1525)
  arc A154 (-395.3933, -1553.1525) -> (-395.3933, -1513.1525) centre (-395.3933, -1533.1525) ccw
  line L145 (-395.3933, -1553.1525) -> (-461.4333, -1553.1525)
  line L146 (-757.7667, -2133.1525) -> (-823.8067, -2133.1525)
  arc A155 (-823.8067, -2093.1525) -> (-823.8067, -2133.1525) centre (-823.8067, -2113.1525) ccw
  line L147 (-823.8067, -2093.1525) -> (-757.7667, -2093.1525)
  arc A156 (-757.7667, -2133.1525) -> (-757.7667, -2093.1525) centre (-757.7667, -2113.1525) ccw
  line L148 (-757.7667, -2353.1525) -> (-823.8067, -2353.1525)
  arc A157 (-823.8067, -2313.1525) -> (-823.8067, -2353.1525) centre (-823.8067, -2333.1525) ccw
  line L149 (-823.8067, -2313.1525) -> (-757.7667, -2313.1525)
  arc A158 (-757.7667, -2353.1525) -> (-757.7667, -2313.1525) centre (-757.7667, -2333.1525) ccw
  line L150 (-757.7667, -1733.1525) -> (-823.8067, -1733.1525)
  arc A159 (-823.8067, -1693.1525) -> (-823.8067, -1733.1525) centre (-823.8067, -1713.1525) ccw
  line L151 (-823.8067, -1693.1525) -> (-757.7667, -1693.1525)
  arc A160 (-757.7667, -1733.1525) -> (-757.7667, -1693.1525) centre (-757.7667, -1713.1525) ccw
  line L152 (-757.7667, -1953.1525) -> (-823.8067, -1953.1525)
  arc A161 (-823.8067, -1913.1525) -> (-823.8067, -1953.1525) centre (-823.8067, -1933.1525) ccw
  line L153 (-823.8067, -1913.1525) -> (-757.7667, -1913.1525)
  arc A162 (-757.7667, -1953.1525) -> (-757.7667, -1913.1525) centre (-757.7667, -1933.1525) ccw
  line L154 (-757.7667, -1333.1525) -> (-823.8067, -1333.1525)
  arc A163 (-823.8067, -1293.1525) -> (-823.8067, -1333.1525) centre (-823.8067, -1313.1525) ccw
  line L155 (-823.8067, -1293.1525) -> (-757.7667, -1293.1525)
  arc A164 (-757.7667, -1333.1525) -> (-757.7667, -1293.1525) centre (-757.7667, -1313.1525) ccw
  line L156 (-757.7667, -1553.1525) -> (-823.8067, -1553.1525)
  arc A165 (-823.8067, -1513.1525) -> (-823.8067, -1553.1525) centre (-823.8067, -1533.1525) ccw
  line L157 (-823.8067, -1513.1525) -> (-757.7667, -1513.1525)
  arc A166 (-757.7667, -1553.1525) -> (-757.7667, -1513.1525) centre (-757.7667, -1533.1525) ccw
  line L158 (-214.2067, -133.1525) -> (-280.2467, -133.1525)
  arc A167 (-280.2467, -93.1525) -> (-280.2467, -133.1525) centre (-280.2467, -113.1525) ccw
  line L159 (-280.2467, -93.1525) -> (-214.2067, -93.1525)
  arc A168 (-214.2067, -133.1525) -> (-214.2067, -93.1525) centre (-214.2067, -113.1525) ccw
  line L160 (-395.3933, -353.1525) -> (-461.4333, -353.1525)
  arc A169 (-461.4333, -313.1525) -> (-461.4333, -353.1525) centre (-461.4333, -333.1525) ccw
  line L161 (-461.4333, -313.1525) -> (-395.3933, -313.1525)
  arc A170 (-395.3933, -353.1525) -> (-395.3933, -313.1525) centre (-395.3933, -333.1525) ccw
  line L162 (-99.06, -493.1525) -> (-33.02, -493.1525)
  arc A171 (-33.02, -533.1525) -> (-33.02, -493.1525) centre (-33.02, -513.1525) ccw
  line L163 (-33.02, -533.1525) -> (-99.06, -533.1525)
  arc A172 (-99.06, -493.1525) -> (-99.06, -533.1525) centre (-99.06, -513.1525) ccw
  line L164 (-99.06, -1113.1525) -> (-33.02, -1113.1525)
  arc A173 (-33.02, -1153.1525) -> (-33.02, -1113.1525) centre (-33.02, -1133.1525) ccw
  line L165 (-33.02, -1153.1525) -> (-99.06, -1153.1525)
  arc A174 (-99.06, -1113.1525) -> (-99.06, -1153.1525) centre (-99.06, -1133.1525) ccw
  arc A175 (-461.4333, -893.1525) -> (-461.4333, -933.1525) centre (-461.4333, -913.1525) ccw
  line L166 (-461.4333, -893.1525) -> (-395.3933, -893.1525)
  arc A176 (-395.3933, -933.1525) -> (-395.3933, -893.1525) centre (-395.3933, -913.1525) ccw
  line L167 (-395.3933, -933.1525) -> (-461.4333, -933.1525)
  line L168 (-576.58, -353.1525) -> (-642.62, -353.1525)
  arc A177 (-642.62, -313.1525) -> (-642.62, -353.1525) centre (-642.62, -333.1525) ccw
  line L169 (-642.62, -313.1525) -> (-576.58, -313.1525)
  arc A178 (-576.58, -353.1525) -> (-576.58, -313.1525) centre (-576.58, -333.1525) ccw
  line L170 (-1186.18, -713.1525) -> (-1120.14, -713.1525)
  arc A179 (-1120.14, -753.1525) -> (-1120.14, -713.1525) centre (-1120.14, -733.1525) ccw
  line L171 (-1120.14, -753.1525) -> (-1186.18, -753.1525)
  arc A180 (-1186.18, -713.1525) -> (-1186.18, -753.1525) centre (-1186.18, -733.1525) ccw
  line L172 (-1120.14, -533.1525) -> (-1186.18, -533.1525)
  arc A181 (-1186.18, -493.1525) -> (-1186.18, -533.1525) centre (-1186.18, -513.1525) ccw
  line L173 (-1186.18, -493.1525) -> (-1120.14, -493.1525)
  arc A182 (-1120.14, -533.1525) -> (-1120.14, -493.1525) centre (-1120.14, -513.1525) ccw
  line L174 (-1186.18, -1113.1525) -> (-1120.14, -1113.1525)
  arc A183 (-1120.14, -1153.1525) -> (-1120.14, -1113.1525) centre (-1120.14, -1133.1525) ccw
  line L175 (-1120.14, -1153.1525) -> (-1186.18, -1153.1525)
  arc A184 (-1186.18, -1113.1525) -> (-1186.18, -1153.1525) centre (-1186.18, -1133.1525) ccw
  line L176 (-1120.14, -933.1525) -> (-1186.18, -933.1525)
  arc A185 (-1186.18, -893.1525) -> (-1186.18, -933.1525) centre (-1186.18, -913.1525) ccw
  line L177 (-1186.18, -893.1525) -> (-1120.14, -893.1525)
  arc A186 (-1120.14, -933.1525) -> (-1120.14, -893.1525) centre (-1120.14, -913.1525) ccw
  line L178 (-576.58, -133.1525) -> (-642.62, -133.1525)
  arc A187 (-642.62, -93.1525) -> (-642.62, -133.1525) centre (-642.62, -113.1525) ccw
  line L179 (-642.62, -93.1525) -> (-576.58, -93.1525)
  arc A188 (-576.58, -133.1525) -> (-576.58, -93.1525) centre (-576.58, -113.1525) ccw
  line L180 (-938.9533, -933.1525) -> (-1004.9933, -933.1525)
  arc A189 (-1004.9933, -893.1525) -> (-1004.9933, -933.1525) centre (-1004.9933, -913.1525) ccw
  line L181 (-1004.9933, -893.1525) -> (-938.9533, -893.1525)
  arc A190 (-938.9533, -933.1525) -> (-938.9533, -893.1525) centre (-938.9533, -913.1525) ccw
  arc A191 (-1004.9933, -1113.1525) -> (-1004.9933, -1153.1525) centre (-1004.9933, -1133.1525) ccw
  line L182 (-1004.9933, -1113.1525) -> (-938.9533, -1113.1525)
  arc A192 (-938.9533, -1153.1525) -> (-938.9533, -1113.1525) centre (-938.9533, -1133.1525) ccw
  line L183 (-938.9533, -1153.1525) -> (-1004.9933, -1153.1525)
  line L184 (-938.9533, -533.1525) -> (-1004.9933, -533.1525)
  arc A193 (-1004.9933, -493.1525) -> (-1004.9933, -533.1525) centre (-1004.9933, -513.1525) ccw
  line L185 (-1004.9933, -493.1525) -> (-938.9533, -493.1525)
  arc A194 (-938.9533, -533.1525) -> (-938.9533, -493.1525) centre (-938.9533, -513.1525) ccw
  arc A195 (-1004.9933, -713.1525) -> (-1004.9933, -753.1525) centre (-1004.9933, -733.1525) ccw
  line L186 (-1004.9933, -713.1525) -> (-938.9533, -713.1525)
  arc A196 (-938.9533, -753.1525) -> (-938.9533, -713.1525) centre (-938.9533, -733.1525) ccw
  line L187 (-938.9533, -753.1525) -> (-1004.9933, -753.1525)
  line L188 (-757.7667, -353.1525) -> (-823.8067, -353.1525)
  arc A197 (-823.8067, -313.1525) -> (-823.8067, -353.1525) centre (-823.8067, -333.1525) ccw
  line L189 (-823.8067, -313.1525) -> (-757.7667, -313.1525)
  arc A198 (-757.7667, -353.1525) -> (-757.7667, -313.1525) centre (-757.7667, -333.1525) ccw
  line L190 (-757.7667, -133.1525) -> (-823.8067, -133.1525)
  arc A199 (-823.8067, -93.1525) -> (-823.8067, -133.1525) centre (-823.8067, -113.1525) ccw
  line L191 (-823.8067, -93.1525) -> (-757.7667, -93.1525)
  arc A200 (-757.7667, -133.1525) -> (-757.7667, -93.1525) centre (-757.7667, -113.1525) ccw
  arc A201 (-461.4333, -1113.1525) -> (-461.4333, -1153.1525) centre (-461.4333, -1133.1525) ccw
  line L192 (-461.4333, -1113.1525) -> (-395.3933, -1113.1525)
  arc A202 (-395.3933, -1153.1525) -> (-395.3933, -1113.1525) centre (-395.3933, -1133.1525) ccw
  line L193 (-395.3933, -1153.1525) -> (-461.4333, -1153.1525)
  line L194 (-280.2467, -493.1525) -> (-214.2067, -493.1525)
  arc A203 (-214.2067, -533.1525) -> (-214.2067, -493.1525) centre (-214.2067, -513.1525) ccw
  line L195 (-214.2067, -533.1525) -> (-280.2467, -533.1525)
  arc A204 (-280.2467, -493.1525) -> (-280.2467, -533.1525) centre (-280.2467, -513.1525) ccw
  arc A205 (-280.2467, -713.1525) -> (-280.2467, -753.1525) centre (-280.2467, -733.1525) ccw
  line L196 (-280.2467, -713.1525) -> (-214.2067, -713.1525)
  arc A206 (-214.2067, -753.1525) -> (-214.2067, -713.1525) centre (-214.2067, -733.1525) ccw
  line L197 (-214.2067, -753.1525) -> (-280.2467, -753.1525)
  line L198 (-395.3933, -133.1525) -> (-461.4333, -133.1525)
  arc A207 (-461.4333, -93.1525) -> (-461.4333, -133.1525) centre (-461.4333, -113.1525) ccw
  line L199 (-461.4333, -93.1525) -> (-395.3933, -93.1525)
  arc A208 (-395.3933, -133.1525) -> (-395.3933, -93.1525) centre (-395.3933, -113.1525) ccw
  arc A209 (-1004.9933, -1513.1525) -> (-1004.9933, -1553.1525) centre (-1004.9933, -1533.1525) ccw
  line L200 (-1004.9933, -1513.1525) -> (-938.9533, -1513.1525)
  arc A210 (-938.9533, -1553.1525) -> (-938.9533, -1513.1525) centre (-938.9533, -1533.1525) ccw
  line L201 (-938.9533, -1553.1525) -> (-1004.9933, -1553.1525)
  line L202 (-938.9533, -1333.1525) -> (-1004.9933, -1333.1525)
  arc A211 (-1004.9933, -1293.1525) -> (-1004.9933, -1333.1525) centre (-1004.9933, -1313.1525) ccw
  line L203 (-1004.9933, -1293.1525) -> (-938.9533, -1293.1525)
  arc A212 (-938.9533, -1333.1525) -> (-938.9533, -1293.1525) centre (-938.9533, -1313.1525) ccw
  arc A213 (-1004.9933, -1913.1525) -> (-1004.9933, -1953.1525) centre (-1004.9933, -1933.1525) ccw
  line L204 (-1004.9933, -1913.1525) -> (-938.9533, -1913.1525)
  arc A214 (-938.9533, -1953.1525) -> (-938.9533, -1913.1525) centre (-938.9533, -1933.1525) ccw
  line L205 (-938.9533, -1953.1525) -> (-1004.9933, -1953.1525)
  line L206 (-938.9533, -1733.1525) -> (-1004.9933, -1733.1525)
  arc A215 (-1004.9933, -1693.1525) -> (-1004.9933, -1733.1525) centre (-1004.9933, -1713.1525) ccw
  line L207 (-1004.9933, -1693.1525) -> (-938.9533, -1693.1525)
  arc A216 (-938.9533, -1733.1525) -> (-938.9533, -1693.1525) centre (-938.9533, -1713.1525) ccw
  arc A217 (-1004.9933, -2313.1525) -> (-1004.9933, -2353.1525) centre (-1004.9933, -2333.1525) ccw
  line L208 (-1004.9933, -2313.1525) -> (-938.9533, -2313.1525)
  arc A218 (-938.9533, -2353.1525) -> (-938.9533, -2313.1525) centre (-938.9533, -2333.1525) ccw
  line L209 (-938.9533, -2353.1525) -> (-1004.9933, -2353.1525)
  line L210 (-938.9533, -2133.1525) -> (-1004.9933, -2133.1525)
  arc A219 (-1004.9933, -2093.1525) -> (-1004.9933, -2133.1525) centre (-1004.9933, -2113.1525) ccw
  line L211 (-1004.9933, -2093.1525) -> (-938.9533, -2093.1525)
  arc A220 (-938.9533, -2133.1525) -> (-938.9533, -2093.1525) centre (-938.9533, -2113.1525) ccw
  line L212 (-99.06, -1513.1525) -> (-33.02, -1513.1525)
  arc A221 (-33.02, -1553.1525) -> (-33.02, -1513.1525) centre (-33.02, -1533.1525) ccw
  line L213 (-33.02, -1553.1525) -> (-99.06, -1553.1525)
  arc A222 (-99.06, -1513.1525) -> (-99.06, -1553.1525) centre (-99.06, -1533.1525) ccw
  arc A223 (-461.4333, -1293.1525) -> (-461.4333, -1333.1525) centre (-461.4333, -1313.1525) ccw
  line L214 (-461.4333, -1293.1525) -> (-395.3933, -1293.1525)
  arc A224 (-395.3933, -1333.1525) -> (-395.3933, -1293.1525) centre (-395.3933, -1313.1525) ccw
  line L215 (-395.3933, -1333.1525) -> (-461.4333, -1333.1525)
  line L216 (-99.06, -1693.1525) -> (-33.02, -1693.1525)
  arc A225 (-33.02, -1733.1525) -> (-33.02, -1693.1525) centre (-33.02, -1713.1525) ccw
  line L217 (-33.02, -1733.1525) -> (-99.06, -1733.1525)
  arc A226 (-99.06, -1693.1525) -> (-99.06, -1733.1525) centre (-99.06, -1713.1525) ccw
  line L218 (-99.06, -2313.1525) -> (-33.02, -2313.1525)
  arc A227 (-33.02, -2353.1525) -> (-33.02, -2313.1525) centre (-33.02, -2333.1525) ccw
  line L219 (-33.02, -2353.1525) -> (-99.06, -2353.1525)
  arc A228 (-99.06, -2313.1525) -> (-99.06, -2353.1525) centre (-99.06, -2333.1525) ccw
  arc A229 (-461.4333, -2093.1525) -> (-461.4333, -2133.1525) centre (-461.4333, -2113.1525) ccw
  line L220 (-461.4333, -2093.1525) -> (-395.3933, -2093.1525)
  arc A230 (-395.3933, -2133.1525) -> (-395.3933, -2093.1525) centre (-395.3933, -2113.1525) ccw
  line L221 (-395.3933, -2133.1525) -> (-461.4333, -2133.1525)
  line L222 (-666.0507, -1047.1575) -> (-731.5763, -1047.1637)
  arc A231 (-731.5761, -1007.1637) -> (-731.5763, -1047.1637) centre (-731.5762, -1027.1637) ccw
  line L223 (-731.5761, -1007.1637) -> (-665.5361, -1007.1642)
  arc A232 (-666.0507, -1047.1575) -> (-665.5361, -1007.1642) centre (-666.0526, -1027.1575) ccw
  arc A233 (-916.5761, -607.1637) -> (-916.5763, -647.1637) centre (-916.5762, -627.1637) ccw
  line L224 (-916.5761, -607.1637) -> (-850.5361, -607.1642)
  arc A234 (-851.0507, -647.1575) -> (-850.5361, -607.1642) centre (-851.0526, -627.1575) ccw
  line L225 (-851.0507, -647.1575) -> (-916.5763, -647.1637)
  line L226 (-183.6639, -607.1642) -> (-117.6239, -607.1637)
  arc A235 (-117.6237, -647.1637) -> (-117.6239, -607.1637) centre (-117.6238, -627.1637) ccw
  line L227 (-117.6237, -647.1637) -> (-183.1493, -647.1575)
  arc A236 (-183.6639, -607.1642) -> (-183.1493, -647.1575) centre (-183.1474, -627.1575) ccw
  arc A237 (-731.5761, -207.1637) -> (-731.5763, -247.1637) centre (-731.5762, -227.1637) ccw
  line L228 (-731.5761, -207.1637) -> (-665.5361, -207.1642)
  arc A238 (-666.0507, -247.1575) -> (-665.5361, -207.1642) centre (-666.0526, -227.1575) ccw
  line L229 (-666.0507, -247.1575) -> (-731.5763, -247.1637)
  line L230 (-368.6639, -1407.1642) -> (-302.6239, -1407.1637)
  arc A239 (-302.6237, -1447.1637) -> (-302.6239, -1407.1637) centre (-302.6238, -1427.1637) ccw
  line L231 (-302.6237, -1447.1637) -> (-368.1493, -1447.1575)
  arc A240 (-368.6639, -1407.1642) -> (-368.1493, -1447.1575) centre (-368.1474, -1427.1575) ccw
  line L232 (-1036.0507, -1447.1575) -> (-1101.5763, -1447.1637)
  arc A241 (-1101.5761, -1407.1637) -> (-1101.5763, -1447.1637) centre (-1101.5762, -1427.1637) ccw
  line L233 (-1101.5761, -1407.1637) -> (-1035.5361, -1407.1642)
  arc A242 (-1036.0507, -1447.1575) -> (-1035.5361, -1407.1642) centre (-1036.0526, -1427.1575) ccw
  line L234 (-666.0507, -1847.1575) -> (-731.5763, -1847.1637)
  arc A243 (-731.5761, -1807.1637) -> (-731.5763, -1847.1637) centre (-731.5762, -1827.1637) ccw
  line L235 (-731.5761, -1807.1637) -> (-665.5361, -1807.1642)
  arc A244 (-666.0507, -1847.1575) -> (-665.5361, -1807.1642) centre (-666.0526, -1827.1575) ccw
  line L236 (-368.6639, -2207.1642) -> (-302.6239, -2207.1637)
  arc A245 (-302.6237, -2247.1637) -> (-302.6239, -2207.1637) centre (-302.6238, -2227.1637) ccw
  line L237 (-302.6237, -2247.1637) -> (-368.1493, -2247.1575)
  arc A246 (-368.6639, -2207.1642) -> (-368.1493, -2247.1575) centre (-368.1474, -2227.1575) ccw
  line L238 (-1036.0507, -2247.1575) -> (-1101.5763, -2247.1637)
  arc A247 (-1101.5761, -2207.1637) -> (-1101.5763, -2247.1637) centre (-1101.5762, -2227.1637) ccw
  line L239 (-1101.5761, -2207.1637) -> (-1035.5361, -2207.1642)
  arc A248 (-1036.0507, -2247.1575) -> (-1035.5361, -2207.1642) centre (-1036.0526, -2227.1575) ccw
  circle A249 centre (-34.29, -2020) radius 17.145
  circle A250 centre (-321.945, -2020) radius 17.145
  circle A251 centre (-609.6, -2020) radius 17.145
  circle A252 centre (-321.945, -420) radius 17.145
  circle A253 centre (-897.255, -2020) radius 17.145
  circle A254 centre (-1184.91, -2020) radius 17.145
  circle A255 centre (-34.29, -420) radius 17.145
  circle A256 centre (-34.29, -2420) radius 17.145
  circle A257 centre (-1184.91, -20) radius 17.145
  circle A258 centre (-321.945, -2420) radius 17.145
  circle A259 centre (-609.6, -2420) radius 17.145
  circle A260 centre (-897.255, -20) radius 17.145
  circle A261 centre (-897.255, -2420) radius 17.145
  circle A262 centre (-321.945, -1220) radius 17.145
  circle A263 centre (-34.29, -1220) radius 17.145
  circle A264 centre (-1184.91, -820) radius 17.145
  circle A265 centre (-897.255, -820) radius 17.145
  circle A266 centre (-609.6, -820) radius 17.145
  circle A267 centre (-34.29, -20) radius 17.145
  circle A268 centre (-1184.91, -2420) radius 17.145
  circle A269 centre (-609.6, -20) radius 17.145
  circle A270 centre (-321.945, -20) radius 17.145
  circle A271 centre (-609.6, -1620) radius 17.145
  circle A272 centre (-897.255, -1620) radius 17.145
  circle A273 centre (-321.945, -1620) radius 17.145
  circle A274 centre (-34.29, -1620) radius 17.145
  circle A275 centre (-34.29, -820) radius 17.145
  circle A276 centre (-1184.91, -420) radius 17.145
  circle A277 centre (-1184.91, -1220) radius 17.145
  circle A278 centre (-897.255, -1220) radius 17.145
  circle A279 centre (-321.945, -820) radius 17.145
  circle A280 centre (-609.6, -1220) radius 17.145
  circle A281 centre (-609.6, -420) radius 17.145
  circle A282 centre (-897.255, -420) radius 17.145
  circle A283 centre (-1184.91, -1620) radius 17.145
  line L240 (0, 0) -> (-1219.2, 0)
  line L241 (-1219.2, 0) -> (-1219.2, -2463.8)
  line L242 (-1219.2, -2463.8) -> (0, -2463.8)
  line L243 (0, -2463.8) -> (0, 0)
  line L244 (0, -2463.8) -> (-1219.2, -2463.8)
  line L245 (-1219.2, -2463.8) -> (-1219.2, -25.4)
  line L246 (-1219.2, -25.4) -> (0, -25.4)
  line L247 (0, -25.4) -> (0, -2463.8)
  dimension "d155" = 2438.4
  dimension "d156" = 1219.2
  constraint horizontal L244
  constraint vertical L245
  constraint horizontal L246
  constraint vertical L247
  constraint coincident L243 L246.end
  constraint tangent A8 L246
  measures "d155" distance of L241.end L245.end
  measures "d156" distance of L242.end L241.end
equation "hexagon = 172 mm + hexagon_fitness"
equation "d2 = ( hexagon / 2 )"
equation "separation = 2 mm"
equation "hexagon_fitness = 0.5 mm"
equation "d12 = hexagon + separation"
equation "d16 = hexagon + separation"
equation "d20 = hexagon + separation"
equation "border = 45 mm"
equation "d23 = border"
equation "d24 = border"
equation "d25 = border"
equation "d26 = -border"
equation "d27 = border"
equation "d28 = border"
equation "d29 = border"
equation "d30 = border"
equation "d31 = border"
equation "d32 = -border"
equation "d33 = border"
equation "d34 = -border"
equation "thickness = 0.5 in"
equation "d36 = -thickness"
equation "d38 = -recess"
equation "recess = 1 mm"
equation "d1 = BoardWidth"
equation "d2_1 = BoardLength"
equation "BoardLength = BoardLengthCount * 1\""
equation "BoardWidth = BoardWidthCount * 1\""
equation "MountFirstRowOffset = 20 mm"
equation "MountFeaturesPerRow = 5" comment "3 for 2' Wide Machines, 5 for 4' Wide Machines"
equation "NumberOfCrossMembers = 7" comment "Don't Change This"
equation "CrossMemberSpacing = 400 mm"
equation "MountCounterBoreDiameter = 1.35 in"